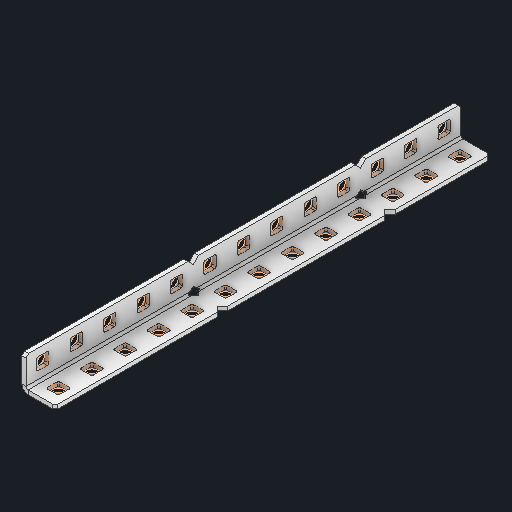
# Autodesk Inventor part: Alu C 1x2x1x35
Saved by Autodesk Inventor 2024 (Build 280153000, 153)
## iProperties
Created: 2022-07-28
Part Number: Alu C 1x2x1x35
Material: Generic
Document SubType Name: Sheet Metal
Designer: ylu12
Density: 1 g/cm^3
Sheet Metal Rule: Default
Appearance: Aluminum
Author: ylu12
Autodesk Inventor part; units mm, degrees
ref_plane "YZ Plane" through (0, 0, 0) normal (1, 0, 0) x (0, 1, 0)
ref_plane "XZ Plane" through (0, 0, 0) normal (0, 1, 0) x (-1, 0, 0)
sketch "Sketch1" plane through (0, 0, 0) normal (0, 1, 0) x (-1, 0, 0)
  line L0 (-6.35, 0) -> (6.35, 0)
  line L1 (6.35, 0) -> (6.35, -165.1)
  line L2 (6.35, -165.1) -> (-6.35, -165.1)
  line L3 (-6.35, -165.1) -> (-6.35, 0)
  line L4 (6.35, 0) -> (-6.35, -165.1) construction
  point P0 (0, 0)
  point P1 (0, 0)
  dimension "d0" = 12.7
  dimension "d1" = 165.1
  constraints: 10 end point, 2 parallel, 1 coincident, 1 horizontal, 1 midpoint, 1 perpendicular
  measures "d0" distance of L1.end L2.end
  measures "d1" distance of L0.end L1.end
extrude "Plate1" add sketch "Sketch1" along normal blind 1.5875
sketch "Sketch2" plane through (-4.7625, 0, 0) normal (-1, 0, 0) x (0, -1, 0)
  line L0 (0, -165.1) -> (0, 0)
  line L1 (0, 0) -> (-12.7, 0)
  line L2 (-12.7, 0) -> (-12.7, -165.1)
  line L3 (-12.7, -165.1) -> (0, -165.1)
  constraints: 6 end point, 1 horizontal, 1 perpendicular, 1 vertical
edge flange "Flanges" height 12.7 angle 90 thickness 1.5875 bend radius 0.7937 thickness toward (-1, 0, 0) relief tear relief width 1.5875 relief depth 0.7937 edges at (-6.35, 1.5875, -82.55) wall of the first edge with corners at (-4.7625, 0, -165.1) (-4.7625, 0, 0) (-4.7625, 12.7, 0) (-4.7625, 12.7, -165.1)
bend "Bend1"
corner "Corner1"
sketch "Sketch8" plane through (0, 0, 0) normal (0, -1, 0) x (1, 0, 0)
  line L0 (6.35, 0) -> (-3.9687, 0) construction
  line L1 (2.9718, -4.0386) -> (-0.635, -4.0386)
  line L2 (-1.143, -4.5466) -> (-1.143, -8.1534)
  line L3 (-0.635, -8.6614) -> (2.9718, -8.6614)
  line L4 (3.4798, -8.1534) -> (3.4798, -4.5466)
  arc A0 (3.4798, -4.5466) -> (2.9718, -4.0386) centre (2.9718, -4.5466) ccw
  arc A1 (2.9718, -8.6614) -> (3.4798, -8.1534) centre (2.9718, -8.1534) ccw
  arc A2 (-1.143, -8.1534) -> (-0.635, -8.6614) centre (-0.635, -8.1534) ccw
  arc A3 (-0.635, -4.0386) -> (-1.143, -4.5466) centre (-0.635, -4.5466) ccw
  line L5 (2.9718, -4.5466) -> (-0.635, -8.1534) construction
  line L6 (6.35, -165.1) -> (6.35, 0) construction
  point P0 (0, 0)
  point P1 (-1.143, -8.6614)
  point P2 (3.4798, -8.6614)
  point P3 (12.7, 0)
  point P4 (1.1684, -6.35)
  dimension "d49" = 4.6228
  dimension "d50" = 0.508
  dimension "d52" = 6.35
  dimension "d123" = 5.1816
  constraints: 10 end point, 8 point on circle, 8 tangent, 4 centre point, 4 point on line, 3 equal radius, 2 parallel, 2 perpendicular, 1 horizontal, 1 midpoint, 1 other
  measures "d49" distance of point (3.48, -8.661) point (-1.143, -8.661)
  measures "d50" radius of A0
  measures "d52" distance from line of L0 point (1.168, -6.35)
extrude "Body Stamp" cut sketch "Sketch8" against normal blind 1.5875
sketch "Sketch9" plane through (0, 0, 0) normal (0, -1, 0) x (1, 0, 0)
  arc A0 (3.4798, -4.5466) -> (2.9718, -4.0386) centre (2.9718, -4.5466) ccw construction
  arc A1 (-1.143, -8.1534) -> (-0.635, -8.6614) centre (-0.635, -8.1534) ccw construction
  line L0 (2.9718, -4.5466) -> (-0.635, -8.1534) construction
  circle A2 centre (1.1684, -6.35) radius 2.1844
  point P0 (0, 0)
  dimension "d55" = 4.3688
  constraints: 2 end point, 1 centre point, 1 midpoint
  measures "d55" diameter of A2
surface extrude "Body Circle" sketch "Sketch9" against normal up to surface (1.5875 mm away) shown yes curves A2
sketch "Body Pattern Sketch" plane through (0, 0, 0) normal (0, -1, 0) x (1, 0, 0)
  line L0 (1.1684, -6.35) -> (1.1684, 0) construction
  circle A0 centre (1.1684, -6.35) radius 2.1844 construction
  point P0 (1.1684, -19.05)
  point P1 (1.1684, -31.75)
  point P2 (1.1684, -44.45)
  point P3 (1.1684, -57.15)
  point P4 (1.1684, -69.85)
  point P5 (1.1684, -82.55)
  point P6 (1.1684, -95.25)
  point P7 (1.1684, -107.95)
  point P8 (1.1684, -120.65)
  point P9 (1.1684, -133.35)
  point P10 (1.1684, -146.05)
  point P11 (1.1684, -158.75)
  dimension "d133" = 12.7
  constraints: 2 end point, 2 vertical, 1 coincident, 12 other
  measures "d133" distance of L0.start point (1.168, -19.05)
pattern_sketch "Body Pattern" of "Body Stamp", "Body Circle" from (1.1684, 0, -6.35) copies at (1.1684, 0, -19.05) at (1.1684, 0, -31.75) at (1.1684, 0, -44.45) at (1.1684, 0, -57.15) at (1.1684, 0, -69.85) at (1.1684, 0, -82.55) at (1.1684, 0, -95.25) at (1.1684, 0, -107.95) at (1.1684, 0, -120.65) at (1.1684, 0, -133.35) at (1.1684, 0, -146.05) at (1.1684, 0, -158.75)
sketch "Arc Length" plane through (19.05, 2.3812, 0) normal (0, 0, 1) x (1, 0, 0)
  line L0 (-25.4, 0) -> (-23.8125, 0) projected
  arc A0 (-25.4, 0) -> (-23.0187, -2.3813) centre (-23.0187, 0) ccw projected
  line L1 (-23.0187, -0.7937) -> (-23.0187, -2.3813) projected
  arc A1 (-23.8125, 0) -> (-23.0187, -0.7937) centre (-23.0187, 0) ccw projected
  point P0 (-19.05, -2.3812)
  dimension "d126" = 1.2468
  dimension "d127" = 3.7405
sketch "Sketch13" plane through (-6.35, 0, 279.4) normal (1, 0, 0) x (0, 0, -1)
  line L0 (340.868, 12.7) -> (342.9, 10.668)
  line L1 (342.9, 10.668) -> (344.932, 12.7)
  line L2 (340.868, 12.7) -> (344.932, 12.7)
  line L3 (342.9, 3.3972) -> (340.6372, 1.1344)
  line L4 (340.6372, 1.1344) -> (342.9, -1.1284)
  line L5 (342.9, -1.1284) -> (345.1628, 1.1344)
  line L6 (345.1628, 1.1344) -> (342.9, 3.3972)
  line L7 (342.9, 3.3972) -> (342.9, -1.1284) construction
  line L8 (342.9, 10.668) -> (342.9, 3.3972) construction
  line L9 (444.5, 12.7) -> (279.4, 12.7) projected
  line L10 (444.5, 2.3813) -> (279.4, 2.3813) construction
  line L11 (279.4, 12.7) -> (279.4, 2.3813) construction
  point P0 (444.5, -11.9062)
  point P1 (279.4, 0)
  dimension "d86" = 4.5256
  dimension "d128" = 2.032
  dimension "d129" = 1.016
  dimension "d130" = 63.5
  constraints: 19 end point, 6 perpendicular, 2 vertical, 1 collinear, 1 other
  measures "d86" distance of L3.start L4.end
  measures "d128" distance from line of L2 L0.end
  measures "d130" distance between parallel lines of L11 L8
cut across bends "Notch" sketch "Sketch13" k factor 0.44
pattern_linear "Notch Pattern" count 2 spacing 63.5 along (0, 0, -1) of "Notch"
ref_plane "Diagonal Plane" through (-4.7625, 1.5875, 0) normal (-0.7071068, 0.7071068, 0) x (0, 0, 1)
mirror "Everything Mirrored" about plane through (-4.7625, 1.5875, 0) normal (-0.7071068, 0.7071068, 0) of "Body Stamp", "Body Circle", "Body Pattern", "Notch", "Notch Pattern"
chamfer "End Chamfer" distance 1.016 angle 45 4 edges at (-5.5562, 12.7, -165.1) (-5.5562, 12.7, 0) (6.35, 0.7937, 0) (6.35, 0.7937, -165.1)
equation "\"d53\" = Thickness"
equation "\"d89\" = Thickness"
equation "\"d1\" = 12.7 * Length"
equation "\"d2\" = Thickness"
equation "\"d3\" = BendReliefWidth"
equation "\"d4\" = BendReliefDepth"
equation "\"d5\" = MinimumRemnant"
equation "\"d6\" = TransitionRadius"
equation "\"d10\" = CornerReliefSize"
equation "\"d11\" = GapSize"
equation "\"d12\" = JacobiRadiusSize"
equation "\"BendRadius\" = Thickness"
equation "\"BendReliefWidth\" = Thickness"
equation "\"BendReliefDepth\" = 0.5 * Thickness"
equation "\"CornerReliefSize\" = 4 * Thickness"
equation "\"MinimumRemnant\" = 2 * Thickness"
equation "\"TransitionRadius\" = BendRadius"
equation "\"JacobiRadiusSize\" = BendRadius"
equation "\"GapSize\" = Thickness"
equation "\"Thickness\" = 1.5875"
equation "\"Length\" = 13"
body "Solid1"
body "Srf91"
body "Srf92"
body "Srf856"
body "Srf857"
body "Srf858"
body "Srf859"
body "Srf860"
body "Srf861"
body "Srf1275"
body "Srf1276"
body "Srf1278"
body "Srf1279"
body "Srf1280"
body "Srf1281"
body "Srf1282"
body "Srf1283"
body "Srf1383"
body "Srf1384"
body "Srf1385"
body "Srf1386"
body "Srf1387"
body "Srf1388"
body "Srf1475"
body "Srf1476"
body "Srf1477"
body "Srf1478"
body "Srf1479"
body "Srf1480"
